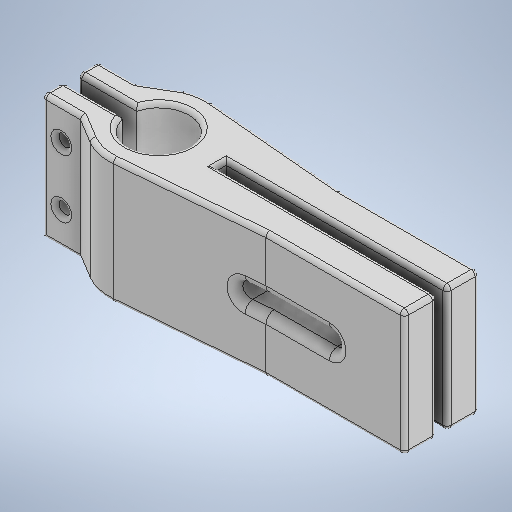
# Autodesk Inventor part: jonction_aile_axe_centrale
Saved by Autodesk Inventor 2025.1 (Build 291241000, 241)
## iProperties
Created: 2025-05-26
Part Number: jonction_aile_axe_centrale
Material: Générique
Document SubType Name: Modeling
Designer: chapuzet
Density: 1 g/cm^3
Appearance: Par défaut
Author: chapuzet
## iProperties of the stored document jonction_aile_axe_centrale_Impression 3D.ipt
Created: 2025-06-04
Part Number: jonction_aile_axe_centrale_Impression 3D
Material: Générique
Document SubType Name: Modeling
Designer: chapuzet
Density: 1 g/cm^3
Appearance: Par défaut
Author: chapuzet
Autodesk Inventor part; units mm, degrees
ref_plane "YZ Plane" through (0, 0, 0) normal (1, 0, 0) x (0, 1, 0)
ref_plane "XZ Plane" through (0, 0, 0) normal (0, 1, 0) x (-1, 0, 0)
ref_plane "XY Plane" through (0, 0, 0) normal (0, 0, 1) x (1, 0, 0)
sketch "Esquisse1" plane through (0, 0, 0) normal (0, 1, 0) x (-1, 0, 0)
  circle A0 centre (0, 0) radius 7.25
  circle A1 centre (0, 0) radius 12
  line L0 (7.25, 11.249) -> (7.25, -11.249)
  line L1 (-30.3619, 0) -> (28.5232, 0)
  line L2 (0, 86.7592) -> (0, -53.8373)
  line L3 (1.4353, 1.75) -> (13.0647, 1.75)
  line L4 (13.0647, 1.75) -> (13.0647, -1.75)
  line L5 (13.0647, -1.75) -> (1.4353, -1.75)
  line L6 (1.4353, -1.75) -> (1.4353, 1.75)
  line L7 (1.4353, 1.75) -> (13.0647, -1.75) construction
  line L8 (13.0647, 1.75) -> (1.4353, -1.75) construction
  line L9 (7.25, 1.75) -> (21.25, 1.75)
  line L10 (21.25, 1.75) -> (21.25, 6.75)
  line L11 (21.25, 6.75) -> (7.25, 6.75)
  line L12 (7.25, 6.75) -> (7.25, 1.75)
  line L13 (7.25, -11.249) -> (7.25, 11.249)
  line L14 (7.25, -1.75) -> (21.25, -1.75)
  line L15 (21.25, -1.75) -> (21.25, -6.75)
  line L16 (21.25, -6.75) -> (7.25, -6.75)
  line L17 (12.0553, 6.75) -> (6.1882, 10.2813)
  line L18 (12.0553, -6.75) -> (4.7887, -11.0031)
  line L19 (-67.9373, 9) -> (-7.9373, 9)
  line L20 (-7.9373, 9) -> (-7.9373, -9)
  line L21 (-7.9373, -9) -> (-67.9373, -9)
  line L22 (-67.9373, -9) -> (-67.9373, 9)
  line L23 (-67.9373, 9) -> (-7.9373, -9) construction
  line L24 (-7.9373, 9) -> (-67.9373, -9) construction
  line L25 (-67.9373, 1.25) -> (-7.9373, 1.25)
  line L26 (-7.9373, 1.25) -> (-7.9373, -1.25)
  line L27 (-7.9373, -1.25) -> (-67.9373, -1.25)
  line L28 (-67.9373, -1.25) -> (-67.9373, 1.25)
  line L29 (-67.9373, 1.25) -> (-7.9373, -1.25) construction
  line L30 (-7.9373, 1.25) -> (-67.9373, -1.25) construction
  line L31 (-14.9373, 9) -> (-14.9373, -9)
  line L32 (-34.7436, 9) -> (-1.048, 11.9541)
  line L33 (-34.7436, -9) -> (-1.048, -11.9541)
  point P0 (7.25, 0)
  point P1 (11.8717, 1.75)
  point P2 (-37.9373, 0)
  point P3 (7.0356, -1.75)
  point P4 (7.0356, 1.75)
  point P5 (-14.9373, 1.25)
  point P6 (-14.9373, -1.25)
  point P7 (-34.7436, -9)
  point P8 (-1.048, -11.9541)
  dimension "d0" = 14.5
  dimension "d1" = 24
  dimension "d2" = 3.5
  dimension "d3" = 14
  dimension "d4" = 5
  dimension "d5" = 5
  dimension "d6" = 14
  dimension "d7" = 9.3783
  dimension "d8" = 18
  dimension "d9" = 60
  dimension "d10" = 2.5
  dimension "d11" = 7
  constraints: 68 end point, 10 point on line, 9 symmetric about line, 8 midpoint, 8 parallel, 5 horizontal, 5 perpendicular, 5 point on circle, 2 coincident, 2 tangent, 2 vertical, 1 centre point, 3 other
  measures "d1" diameter of A1
  measures "d2" distance of L3.end L4.end
  measures "d3" distance of L10.end L11.end
  measures "d4" distance of L9.end L10.end
  measures "d5" distance of L15.start L16.start
  measures "d6" distance of L16.start L16.end
  measures "d7" distance from line of A1.start L10
  measures "d8" distance of L21.end L19.start
  measures "d9" distance of L20.end L21.end
  measures "d10" distance between parallel lines of L27 L25
  measures "d11" distance between parallel lines of L20 L31
extrude "Extrusion1" add sketch "Esquisse1" along normal blind 30 contours A0 L2 A1 L0 L3 | L5 L0 L18 A1 L2 A0 | L0 L11 A1 L3 | L5 A1 L16 L0 | A0 L1 L20 A1 L2 | L2 A1 L20 L1 A0 | L0 A1 L11 | A1 L11 L10 L9 L3 | L16 A1 L0 | L5 L14 L15 L16 A1 | L0 L17 L11 A1 | A1 L17 L0 | A1 L16 L18 | L20 L27 A1 L1 | L1 A1 L25 L20 | A1 L19 L32 | L33 L21 A1 | L1 L31 L25 A1 | A1 L27 L31 L1 | L25 A1 L20 | L20 A1 L27 | A1 L25 L31 L19 | L19 L31 L25 L22 | L21 L31 L27 A1 | L21 L22 L27 L31
sketch "Esquisse2" plane through (0, 0, 0) normal (0, 0, 1) x (1, 0, 0)
  line L0 (-21.25, 0) -> (-21.25, 30) projected
  line L1 (14.9373, 0) -> (67.9373, 0) projected
  line L2 (-21.25, 30) -> (67.9373, 30)
  line L3 (67.9373, 30) -> (67.9373, 0)
  line L4 (67.9373, 0) -> (-21.25, 0)
  line L5 (-21.25, 0) -> (-21.25, 30)
  line L6 (0, 30) -> (0, 0)
  line L7 (-12.0553, 0) -> (-12.0553, 30) projected
  line L8 (-12.0553, 30) -> (-12.0553, 0)
  line L9 (-7.0356, 30) -> (-21.25, 30) projected
  line L10 (-21.25, 30) -> (-12.0553, 30)
  line L11 (-12.0553, 30) -> (-12.0553, 0)
  line L12 (-12.0553, 0) -> (-21.25, 0)
  line L13 (-21.25, 0) -> (-21.25, 30)
  circle A0 centre (-16.6527, 22) radius 1.5
  line L14 (14.9373, 0) -> (14.9373, 30) projected
  line L15 (14.9373, 30) -> (67.9373, 30)
  line L16 (67.9373, 30) -> (67.9373, 0)
  line L17 (67.9373, 0) -> (14.9373, 0)
  line L18 (14.9373, 0) -> (14.9373, 30)
  line L19 (67.9373, 0) -> (67.9373, 30) projected
  line L20 (67.9373, 15) -> (-21.25, 15)
  circle A1 centre (49.9373, 15) radius 2
  circle A2 centre (29.9373, 15) radius 2
  line L21 (29.9373, 17) -> (49.9373, 17)
  line L22 (49.9373, 13) -> (29.9373, 13)
  line L23 (-21.25, 30) -> (-12.0553, 30)
  line L24 (-12.0553, 30) -> (-12.0553, 0)
  line L25 (-12.0553, 0) -> (-21.25, 0)
  line L26 (-21.25, 0) -> (-21.25, 30)
  line L27 (-16.6527, 0) -> (-16.6527, 30)
  circle A3 centre (-16.6527, 8) radius 1.5
  dimension "d14" = 3
  dimension "d15" = 35
  dimension "d16" = 15
  dimension "d17" = 4
  dimension "d22" = 8
  dimension "d23" = 8
  dimension "d24" = 14
  constraints: 44 end point, 8 parallel, 5 perpendicular, 5 point on line, 4 centre point, 4 horizontal, 4 midpoint, 4 point on circle, 3 tangent, 2 equal radius, 1 vertical
  measures "d14" diameter of A0
  measures "d15" distance from line of L14 A1.centre
  measures "d16" distance from line of L14 A2.centre
  measures "d17" diameter of A2
  measures "d22" distance from line of L9 A0.centre
  measures "d23" distance from line of L4 A3.centre
  measures "d24" distance of A0.centre A3.centre
extrude "Extrusion2" cut sketch "Esquisse2" along normal mid plane 30 contours A3 L27 | L27 A3 | L27 A0 | A0 L27 | A2 L20 | L20 A2 | A2 L21 A1 L20 | L20 A1 L22 A2 | A1 L20 | L20 A1
fillet "Congé1" radius 1 52 edges at (67.9373, 15, -9) (67.9373, 15, -1.25) (67.9373, 15, 1.25) (67.9373, 15, 9) (51.3404, 0, 9) (51.3404, 30, 9) (-2.7028, 30, 11.6917) (-9.1218, 30, 8.5157) (17.8958, 30, 10.4771) (-2.7028, 0, 11.6917) (-9.1218, 0, 8.5157) (17.8958, 0, 10.4771) (41.4373, 0, -1.25) (41.4373, 0, 1.25) (14.9373, 0, 0) (-1.9298, 0, -11.8438) (17.8958, 0, -10.4771) (51.3404, 0, -9) (67.9373, 0, 5.125) (67.9373, 0, -5.125) (67.9373, 30, -5.125) (67.9373, 30, 5.125) (51.3404, 30, -9) (41.4373, 30, -1.25) (41.4373, 30, 1.25) (-1.9298, 30, -11.8438) (17.8958, 30, -10.4771) (14.9373, 30, 0) (-8.422, 30, -8.8766) (-16.6527, 30, -6.75) (-16.6527, 30, 6.75) (-14.1428, 30, 1.75) (-14.1428, 30, -1.75) (7.25, 30, 0) (-21.25, 15, -1.75) (-21.25, 15, 1.75) (-21.25, 15, 6.75) (-21.25, 30, 4.25) (-21.25, 30, -4.25) (-21.25, 15, -6.75) (-4.7887, 15, -11.0031) (-8.422, 0, -8.8766) (-16.6527, 0, -6.75) (-21.25, 0, -4.25) (-14.1428, 0, -1.75) (-14.1428, 0, 1.75) (-16.6527, 0, 6.75) (7.25, 0, 0) (-18.1527, 22, 6.75) (-18.1527, 22, -6.75) (-18.1527, 8, 6.75) (-18.1527, 8, -6.75)
fillet "Congé2" radius 2 12 edges at (51.9373, 15, -9) (42.3404, 17, -9) (42.3404, 13, -9) (32.3404, 13, -9.2107) (32.3404, 17, -9.2107) (27.9373, 15, -9.5967) (51.9373, 15, 9) (42.3404, 17, 9) (42.3404, 13, 9) (27.9373, 15, 9.5967) (32.3404, 17, 9.2107) (32.3404, 13, 9.2107)
